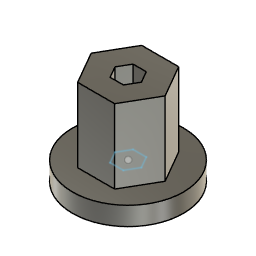
Makita HR2740 Support Extender 3cm (Autodesk Fusion 360 design; units mm, degrees)
Autodesk Fusion 360 part; units mm, degrees
sketch "Sketch1" plane through (0, 0, 0) normal (0, 0, 1) x (1, 0, 0)
  circle A0 centre (0, 0) radius 15
  dimension "d1" = 30
  constraint coincident A0.centre origin
  measures "d1" diameter of A0
extrude "Extrude1" add sketch "Sketch1" along normal blind 5 makes body 1
sketch "Sketch2" plane through (0, 0, 5) normal (0, 0, 1) x (-1, 0, 0)
  circle A0 centre (0, 0) radius 15
  line L0 (5, -8.7) -> (10, -0.0397)
  line L1 (10, -0.0397) -> (5, 8.6205)
  line L2 (5, 8.6205) -> (-5, 8.6205)
  line L3 (-5, 8.6205) -> (-10, -0.0397)
  line L4 (-10, -0.0397) -> (-5, -8.7)
  line L5 (-5, -8.7) -> (5, -8.7)
  point P0 (0, -0.0397)
extrude "Extrude2" add sketch "Sketch2" along normal blind 20 contours L0 L1 L2 L3 L4 L5 bodies 1
sketch "Sketch3" plane through (0, 0, 5) normal (0, 0, 1) x (-1, 0, 0)
  line L0 (1.7898, -3.1538) -> (3.5796, -0.0538)
  line L1 (3.5796, -0.0538) -> (1.7898, 3.0462)
  line L2 (1.7898, 3.0462) -> (-1.7898, 3.0462)
  line L3 (-1.7898, 3.0462) -> (-3.5796, -0.0538)
  line L4 (-3.5796, -0.0538) -> (-1.7898, -3.1538)
  line L5 (-1.7898, -3.1538) -> (1.7898, -3.1538)
  point P0 (0, -0.0538)
  dimension "d6" = 6.2
  measures "d6" distance of L0 L3
extrude "Extrude3" add sketch "Sketch3" along normal blind 14 separate body makes body 2
extrude "Extrude4" add 1 faces at (-0.5966, -0.9795, 19) along direction (0, 0, 1) blind 8 on bodies 2 bodies 2
extrude "Extrude5" cut 1 faces at (-0.5966, -0.9795, 27) along direction (0, 0, -1) blind 19 on bodies 2 bodies 1 2
